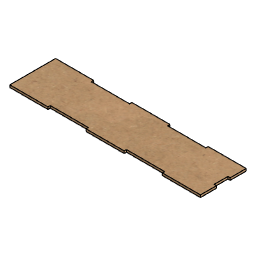
Steps v4 (Autodesk Fusion 360 archive; units mm, degrees)
design "step front"
Autodesk Fusion 360 part; units mm, degrees
sketch "Sketch1" plane through (0, 0, 0) normal (0, 0, 1) x (1, 0, 0) in component "Step front"
  line L0 (125, 30) -> (-125, 30)
  line L1 (-125, 30) -> (-125, -30)
  line L2 (-125, -30) -> (125, -30)
  line L3 (125, -30) -> (125, 30)
  line L4 (125, 30) -> (-125, -30) construction
  line L5 (-125, 30) -> (125, -30) construction
  line L6 (-125, 30) -> (-75, 30)
  line L7 (-75, 30) -> (-75, 27)
  line L8 (-75, 27) -> (-125, 27)
  line L9 (-125, 27) -> (-125, 30)
  line L10 (-25, 27) -> (-75, 27)
  line L11 (-25, 30) -> (-25, 27)
  line L12 (-75, 30) -> (-25, 30)
  line L13 (-75, 30) -> (-75, -30)
  line L14 (25, 27) -> (-25, 27)
  line L15 (25, 30) -> (25, 27)
  line L16 (-25, 30) -> (25, 30)
  line L17 (-25, 30) -> (-25, -30)
  line L18 (75, 27) -> (25, 27)
  line L19 (75, 30) -> (75, 27)
  line L20 (25, 30) -> (75, 30)
  line L21 (25, 30) -> (25, -30)
  line L22 (125, 27) -> (75, 27)
  line L23 (125, 30) -> (125, 27)
  line L24 (75, 30) -> (125, 30)
  line L25 (75, 30) -> (75, -30)
  line L26 (-75, -30) -> (-125, -30)
  line L27 (-75, -27) -> (-75, -30)
  line L28 (-125, -27) -> (-75, -27)
  line L29 (-125, -27) -> (-125, -30)
  line L30 (-25, -30) -> (-75, -30)
  line L31 (-25, -27) -> (-25, -30)
  line L32 (-75, -27) -> (-25, -27)
  line L33 (-75, -27) -> (-75, -30)
  line L34 (25, -30) -> (-25, -30)
  line L35 (25, -27) -> (25, -30)
  line L36 (-25, -27) -> (25, -27)
  line L37 (-25, -27) -> (-25, -30)
  line L38 (75, -30) -> (25, -30)
  line L39 (75, -27) -> (75, -30)
  line L40 (25, -27) -> (75, -27)
  line L41 (25, -27) -> (25, -30)
  line L42 (125, -30) -> (75, -30)
  line L43 (125, -27) -> (125, -30)
  line L44 (75, -27) -> (125, -27)
  line L45 (75, -27) -> (75, -30)
  dimension "d1" = 250
  dimension "d2" = 60
  dimension "d9" = 50
  dimension "d10" = 3
  constraint horizontal L0
  constraint perpendicular L0 L1
  constraint parallel L0 L2
  constraint parallel L1 L3
  constraint coincident L4 origin
  constraint coincident L5 origin
  constraint horizontal L6
  constraint vertical L7
  constraint horizontal L8
  constraint vertical L9
  measures "d1" distance of L1.end L2.end
  measures "d2" distance of L0.end L1.end
  measures "d9" distance of L0.end L6.end
  measures "d10" distance of L0.end L8.end
extrude "Extrude3" add sketch "Sketch1" along normal blind 3 contours L0 L3 L19 L22 L23 L24 L25 | L3 L22 L25 L44 | L0 L11 L14 L15 L16 L17 L21 | L18 L21 L25 L40 | L2 L3 L25 L39 L42 L43 L44 L45 | L14 L17 L21 L36 | L0 L1 L6 L7 L8 L9 L13 | L10 L13 L17 L32 | L2 L17 L21 L31 L34 L35 L36 L37 L41 | L1 L8 L13 L28 | L1 L2 L13 L26 L27 L28 L29 L33 in component "Step front"
sketch "Sketch3" plane through (0, 0, 3) normal (0, 0, 1) x (-1, 0, 0) in component "Step front"
  line L0 (-25, 27) -> (-75, 27)
  line L1 (-75, 27) -> (-75, 30)
  line L2 (-75, 30) -> (-125, 30)
  line L3 (-125, 30) -> (-125, -30)
  line L4 (-125, -30) -> (-75, -30)
  line L5 (-75, -30) -> (-75, -27)
  line L6 (-75, -27) -> (-25, -27)
  line L7 (-25, -27) -> (-25, -30)
  line L8 (-25, -30) -> (25, -30)
  line L9 (25, -30) -> (25, -27)
  line L10 (25, -27) -> (75, -27)
  line L11 (75, -27) -> (75, -30)
  line L12 (75, -30) -> (125, -30)
  line L13 (125, -30) -> (125, 30)
  line L14 (125, 30) -> (75, 30)
  line L15 (75, 30) -> (75, 27)
  line L16 (75, 27) -> (25, 27)
  line L17 (25, 27) -> (25, 30)
  line L18 (25, 30) -> (-25, 30)
  line L19 (-25, 30) -> (-25, 27)
  line L20 (-125, -30) -> (-122, -30) construction
  line L21 (-122, -30) -> (-122, -8) construction
  line L22 (-122, -8) -> (-125, -8) construction
  line L23 (-125, -8) -> (-125, -30) construction
  line L24 (-125, 30) -> (-122, 30) construction
  line L25 (-122, 30) -> (-122, 8) construction
  line L26 (-122, 8) -> (-125, 8) construction
  line L27 (-125, 8) -> (-125, 30) construction
  line L28 (-125, -9) -> (-122, -9)
  line L29 (-122, -9) -> (-122, 9)
  line L30 (-122, 9) -> (-125, 9)
  line L31 (-125, 9) -> (-125, -9)
  dimension "d17" = 22
  dimension "d18" = 3
  dimension "d19" = 22
  constraint horizontal L20
  constraint vertical L21
  constraint horizontal L22
  constraint vertical L23
  constraint coincident L3.end L4.start
  constraint horizontal L24
  constraint vertical L25
  constraint horizontal L26
  constraint vertical L27
  constraint coincident L2.end L3.start
  constraint horizontal L28
  constraint vertical L29
  constraint horizontal L30
  constraint vertical L31
  constraint coincident L25 L29.end
  constraint coincident L3 L28.start
  measures "d17" distance of L3.end L22.end
  measures "d18" distance of L2.end L24.end
  measures "d19" distance of L2.end L26.end
extrude "Extrude4" cut sketch "Sketch3" against normal blind 12 contours L3 L28 L29 L30 L31 in component "Step front"
component "Step front" placed x (1, 0, 0) y (0, 1, 0) z (0, 0, 1) at (0, 0, 0)

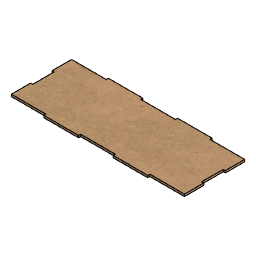
design "Step top"
Autodesk Fusion 360 part; units mm, degrees
sketch "Sketch1" plane through (0, 0, 0) normal (0, 0, 1) x (1, 0, 0)
  line L0 (125, 46.5) -> (-125, 46.5)
  line L1 (-125, 46.5) -> (-125, -46.5)
  line L2 (-125, -46.5) -> (125, -46.5)
  line L3 (125, -46.5) -> (125, 46.5)
  line L4 (125, 46.5) -> (-125, -46.5) construction
  line L5 (-125, 46.5) -> (125, -46.5) construction
  line L6 (-125, 46.5) -> (-75, 46.5)
  line L7 (-75, 46.5) -> (-75, 43.5)
  line L8 (-75, 43.5) -> (-125, 43.5)
  line L9 (-125, 43.5) -> (-125, 46.5)
  line L10 (25, 43.5) -> (-25, 43.5)
  line L11 (-25, 46.5) -> (25, 46.5)
  line L12 (25, 46.5) -> (25, 43.5)
  line L13 (-25, 43.5) -> (-25, 46.5)
  line L14 (125, 43.5) -> (75, 43.5)
  line L15 (75, 46.5) -> (125, 46.5)
  line L16 (125, 46.5) -> (125, 43.5)
  line L17 (75, 43.5) -> (75, 46.5)
  line L18 (-75, -46.5) -> (-125, -46.5)
  line L19 (-125, -43.5) -> (-75, -43.5)
  line L20 (-75, -43.5) -> (-75, -46.5)
  line L21 (-125, -46.5) -> (-125, -43.5)
  line L22 (25, -46.5) -> (-25, -46.5)
  line L23 (-25, -43.5) -> (25, -43.5)
  line L24 (25, -43.5) -> (25, -46.5)
  line L25 (-25, -46.5) -> (-25, -43.5)
  line L26 (125, -46.5) -> (75, -46.5)
  line L27 (75, -43.5) -> (125, -43.5)
  line L28 (125, -43.5) -> (125, -46.5)
  line L29 (75, -46.5) -> (75, -43.5)
  dimension "d1" = 250
  dimension "d2" = 93
  dimension "d13" = 50
  dimension "d14" = 3
  dimension "d17" = 200
  dimension "d18" = -90
  constraint horizontal L0
  constraint perpendicular L0 L1
  constraint parallel L0 L2
  constraint parallel L1 L3
  constraint coincident L4 origin
  constraint coincident L5 origin
  constraint horizontal L6
  constraint vertical L7
  constraint horizontal L8
  constraint vertical L9
  measures "d1" distance of L1.end L2.end
  measures "d2" distance of L0.end L1.end
  measures "d13" distance of L0.end L6.end
  measures "d14" distance of L0.end L8.end
extrude "Extrude3" add sketch "Sketch1" along normal blind 3 contours L0 L1 L2 L3 L7 L8 L10 L12 L13 L14 L17 L19 L20 L23 L24 L25 L27 L29
sketch "Sketch3" plane through (0, 0, 3) normal (0, 0, 1) x (-1, 0, 0)
  line L0 (-75, 46.5) -> (-75, 43.5)
  line L1 (-75, 43.5) -> (-125, 43.5)
  line L2 (-125, 43.5) -> (-125, -43.5)
  line L3 (-125, -43.5) -> (-75, -43.5)
  line L4 (-75, -43.5) -> (-75, -46.5)
  line L5 (-75, -46.5) -> (-25, -46.5)
  line L6 (-25, -46.5) -> (-25, -43.5)
  line L7 (-25, -43.5) -> (25, -43.5)
  line L8 (25, -43.5) -> (25, -46.5)
  line L9 (25, -46.5) -> (75, -46.5)
  line L10 (75, -46.5) -> (75, -43.5)
  line L11 (75, -43.5) -> (125, -43.5)
  line L12 (125, -43.5) -> (125, 43.5)
  line L13 (125, 43.5) -> (75, 43.5)
  line L14 (75, 43.5) -> (75, 46.5)
  line L15 (75, 46.5) -> (25, 46.5)
  line L16 (25, 46.5) -> (25, 43.5)
  line L17 (25, 43.5) -> (-25, 43.5)
  line L18 (-25, 43.5) -> (-25, 46.5)
  line L19 (-25, 46.5) -> (-75, 46.5)
  line L20 (-121.1564, -43.5) -> (-121.1564, -15.5) construction
  line L21 (-121.1564, 43.5) -> (-121.1564, 15.5) construction
  line L22 (-125, -15.5) -> (-122, -15.5)
  line L23 (-122, -15.5) -> (-122, 15.5)
  line L24 (-122, 15.5) -> (-125, 15.5)
  line L25 (-125, 15.5) -> (-125, -15.5)
  dimension "d21" = 28
  dimension "d22" = 28
  dimension "d23" = 3
  dimension "d24" = 31
  constraint coincident L3 L20.start
  constraint perpendicular L3 L20
  constraint coincident L1 L21.start
  constraint perpendicular L1 L21
  constraint horizontal L22
  constraint vertical L23
  constraint horizontal L24
  constraint vertical L25
  constraint coincident L2 L22.start
  measures "d21" distance of L20.start L20.end
  measures "d22" distance of L21.start L21.end
  measures "d23" distance of L22.start L22.end
  measures "d24" distance of L22.start L24.end
extrude "Extrude4" cut sketch "Sketch3" against normal blind 6 contours L2 L22 L23 L24 L25
mirror "Mirror1" about plane through (0, 0, 0) normal (1, 0, 0) of "Extrude4"

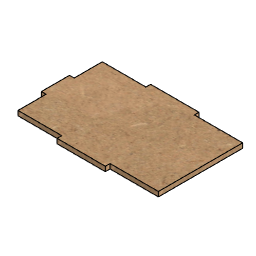
design "side step"
Autodesk Fusion 360 part; units mm, degrees
sketch "Sketch1" plane through (0, 0, 0) normal (0, 0, 1) x (1, 0, 0)
  line L0 (-46.5, 30) -> (46.5, 30)
  line L1 (46.5, 30) -> (46.5, -30)
  line L2 (46.5, -30) -> (-46.5, -30)
  line L3 (-46.5, -30) -> (-46.5, 30)
  line L4 (-46.5, 30) -> (46.5, -30) construction
  line L5 (46.5, 30) -> (-46.5, -30) construction
  line L6 (-46.5, 30) -> (-15.5, 30)
  line L7 (-15.5, 30) -> (-15.5, 27)
  line L8 (-15.5, 27) -> (-46.5, 27)
  line L9 (-46.5, 27) -> (-46.5, 30)
  line L10 (-46.5, -30) -> (-15.5, -30)
  line L11 (-15.5, -30) -> (-15.5, -27)
  line L12 (-15.5, -27) -> (-46.5, -27)
  line L13 (-46.5, -27) -> (-46.5, -30)
  line L14 (46.5, 30) -> (15.5, 30)
  line L15 (15.5, 30) -> (15.5, 27)
  line L16 (15.5, 27) -> (46.5, 27)
  line L17 (46.5, 27) -> (46.5, 30)
  line L18 (46.5, -30) -> (15.5, -30)
  line L19 (15.5, -30) -> (15.5, -27)
  line L20 (15.5, -27) -> (46.5, -27)
  line L21 (46.5, -27) -> (46.5, -30)
  line L22 (46.5, 30) -> (43.5, 30)
  line L23 (43.5, 30) -> (43.5, 27)
  line L24 (43.5, 27) -> (46.5, 27)
  line L25 (46.5, 27) -> (46.5, 30)
  line L26 (46.5, -30) -> (43.5, -30)
  line L27 (43.5, -30) -> (43.5, -27)
  line L28 (43.5, -27) -> (46.5, -27)
  line L29 (46.5, -27) -> (46.5, -30)
  line L30 (-46.5, 27) -> (-43.5, 27)
  line L31 (-43.5, 27) -> (-43.5, 9)
  line L32 (-43.5, 9) -> (-46.5, 9)
  line L33 (-46.5, 9) -> (-46.5, 27)
  line L34 (-46.5, -27) -> (-43.5, -27)
  line L35 (-43.5, -27) -> (-43.5, -9)
  line L36 (-43.5, -9) -> (-46.5, -9)
  line L37 (-46.5, -9) -> (-46.5, -27)
  dimension "d1" = 93
  dimension "d2" = 60
  dimension "d3" = 31
  dimension "d4" = 3
  dimension "d5" = 31
  dimension "d6" = 3
  dimension "d7" = 31
  dimension "d8" = 3
  dimension "d9" = 31
  dimension "d10" = 3
  dimension "d11" = 3
  dimension "d12" = 3
  dimension "d13" = 3
  dimension "d14" = 3
  dimension "d15" = 3
  dimension "d16" = 18
  dimension "d17" = 3
  dimension "d18" = 18
  constraint horizontal L0
  constraint perpendicular L0 L1
  constraint parallel L0 L2
  constraint parallel L1 L3
  constraint coincident L4 origin
  constraint coincident L5 origin
  constraint horizontal L6
  constraint vertical L7
  constraint horizontal L8
  constraint vertical L9
  constraint horizontal L10
  constraint vertical L11
  constraint horizontal L12
  constraint vertical L13
  constraint horizontal L14
  constraint vertical L15
  constraint horizontal L16
  constraint vertical L17
  constraint horizontal L18
  constraint vertical L19
  constraint horizontal L20
  constraint vertical L21
  constraint horizontal L22
  constraint vertical L23
  constraint horizontal L24
  constraint vertical L25
  constraint horizontal L26
  constraint vertical L27
  constraint horizontal L28
  constraint vertical L29
  constraint horizontal L30
  constraint vertical L31
  constraint horizontal L32
  constraint vertical L33
  constraint horizontal L34
  constraint vertical L35
  constraint horizontal L36
  constraint vertical L37
  measures "d1" distance of L1.end L2.end
  measures "d2" distance of L0.end L1.end
  measures "d3" distance of L0.start L6.end
  measures "d4" distance of L0.start L8.end
  measures "d5" distance of L2.end L10.end
  measures "d6" distance of L2.end L12.end
  measures "d7" distance of L0.end L14.end
  measures "d8" distance of L0.end L16.end
  measures "d9" distance of L1.end L18.end
  measures "d10" distance of L1.end L20.end
  measures "d11" distance of L0.end L22.end
  measures "d12" distance of L0.end L16.end
  measures "d13" distance of L1.end L26.end
  measures "d14" distance of L1.end L20.end
  measures "d15" distance of L8.end L30.end
  measures "d16" distance of L8.end L32.end
  measures "d17" distance of L12.end L34.end
  measures "d18" distance of L12.end L36.end
extrude "Extrude1" add sketch "Sketch1" along normal blind 3 contours L0 L1 L2 L3 L7 L8 L11 L12 L15 L16 L19 L20 L24 L28 L31 L32 L35 L36
